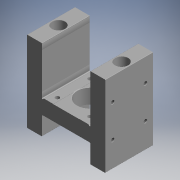
# Autodesk Inventor part: 2608532 EAGF-V2-KF-100---(F)
Saved by Autodesk Inventor 2017.3 (Build 213256000, 256)
## iProperties
Part Number: 2608532 EAGF-V2-KF-100---(F)
Material: Generic
Catalog Web Link: www.cadenas.de
Description: EAGF-(F)-Guide
Vendor: FESTO
Document SubType Name: Modeling
Designer: partserver
Manufacturer: FESTO
Mass: 2427.58 g
Surface Area: 2629 cm^2
Volume: 2427.58 cm^3
Density: 1 g/cm^3
Appearance: PSOLRGB-192-192-192
Category: PARTsolutions
Company: FESTO
Title: 2608532 EAGF-V2-KF-100---(F)
Author: Cadenas PARTsolutions
Comments: Guide
PSOL_IDENT_0: {$CADENAS_DATA\23d-libs\festo\parts\e\eagf\parts\eagf_fuehr.prj},198 {VTYP=3D},{NB=2608532 EAGF-V2-K
PSOL_IDENT_1: F-100---(F)},{LINA=2608532 EAGF-V2-KF-100---(F)},{NN=EAGF-(F)},{DATE=22.07.2021 15:11:35},{GEOMDATE=
PSOL_IDENT_2: 14.04.2021 08:28:38},{VERSION=},{LINEID=30},{WBVAR=},{WBNUMERIC=}  {NB=2608532 EAGF-V2-KF-100---(F)}
PSOL_IDENT_3: ,{LINA=2608532 EAGF-V2-KF-100---(F)},{KT=DUMMY},{TNR=2608532},{TYP=EAGF-V2-KF-100},{KDM=100},{B1=213
PSOL_IDENT_4: .000},{B2=132.000},{B3=70.000},{B4=172.000},{B5=150.000},{D1=35.000},{D2=33.000},{D4=70.000},{D5=18.
PSOL_IDENT_5: 000},{D6=11.000},{D7=10.000},{H1=130.000},{H2=89.000},{H3=65.000},{L1=220.000},{L2=41.000},{L3=128.0
PSOL_IDENT_6: 00},{L4=89.000},{L5=0.000},{L6=24.500},{L7=112.900},{L8=0.000},{T1=0.500},{T2=45.000},{T3=6.000},{T4=
PSOL_IDENT_7: 20.000},{T5=24.000},{F=1.500},{L2J=127.000},{LR1=0.000},{LR2=0.000},{LR3=0.000},{T6=0.000},{LL1=0.00
PSOL_IDENT_8: 0},{LL2=0.000},{LL3=0.000},{LL4=0.000},{LL5=0.000},{TG=89.000}
NB: 2608532 EAGF-V2-KF-100---(F)
NN: EAGF-(F)
NT: Guide
NBSYN: $TNR. $TYP.---(F)
LINA: 2608532 EAGF-V2-KF-100---(F)
CATALOG: Festo
TNR: 2608532
TYP: EAGF-V2-KF-100
KDM: 100
B1: 213
B2: 132
B3: 70
B4: 172
B5: 150
D1: 35
D2: 33
D4: 70
D5: 18
D6: 11
D7: 10
H1: 130
H2: 89
H3: 65
L1: 220
L2: 41
L3: 128
L4: 89
L5: 0
L6: 24.5
L7: 112.9
L8: 0
T1: 0.5
T2: 45
T3: 6
T4: 20
T5: 24
F: 1.5
L2J: 127
LR1: 0
LR2: 0
LR3: 0
T6: 0
LL1: 0
LL2: 0
LL3: 0
LL4: 0
LL5: 0
TG: 89
SUPPLIER: FESTO
ARTICLENO: 2608532 EAGF-V2-KF-100---(F)
BOMINFO: 2608532 EAGF-V2-KF-100---(F)
CREATOR: CADENAS GmbH
Autodesk Inventor part; units mm, degrees
sketch "Sketch_2" plane through (0, 0, 0) normal (0, 1, 0) x (-1, 0, 0)
  arc A0 (106.5, 91) -> (105.5, 92) centre (105.5, 91) ccw
  line L0 (105.5, 92) -> (67, 92)
  arc A1 (67, 92) -> (66, 91) centre (67, 91) ccw
  line L1 (66, 91) -> (66, 43.5)
  arc A2 (63.5, 41) -> (66, 43.5) centre (63.5, 43.5) ccw
  line L2 (63.5, 41) -> (-63.5, 41)
  arc A3 (-66, 43.5) -> (-63.5, 41) centre (-63.5, 43.5) ccw
  line L3 (-66, 43.5) -> (-66, 91)
  arc A4 (-66, 91) -> (-67, 92) centre (-67, 91) ccw
  line L4 (-67, 92) -> (-105.5, 92)
  arc A5 (-105.5, 92) -> (-106.5, 91) centre (-105.5, 91) ccw
  line L5 (-106.5, 91) -> (-106.5, -127)
  arc A6 (-106.5, -127) -> (-105.5, -128) centre (-105.5, -127) ccw
  line L6 (-105.5, -128) -> (-67, -128)
  arc A7 (-67, -128) -> (-66.0931, -126.5786) centre (-67, -127) ccw
  arc A8 (-66.0931, -126.5786) -> (-66, -111.8466) centre (-115.5, -118.9) ccw
  line L7 (-66, -111.8466) -> (-66, -13.0534)
  arc A9 (-66, -13.0534) -> (-65.9994, 1.0491) centre (-115.5, -6) ccw
  arc A10 (-62.0635, 1.5) -> (-65.9994, 1.0491) centre (-64, 1) ccw
  arc A11 (-62.0635, 1.5) -> (-60.127, 0) centre (-60.127, 2) ccw
  line L8 (-60.127, 0) -> (-35, 0)
  line L9 (-35, 0) -> (-35, 0.5)
  line L10 (-35, 0.5) -> (35, 0.5)
  line L11 (35, 0.5) -> (35, 0)
  line L12 (35, 0) -> (60.127, 0)
  arc A12 (60.127, 0) -> (62.0635, 1.5) centre (60.127, 2) ccw
  arc A13 (65.9994, 1.0491) -> (62.0635, 1.5) centre (64, 1) ccw
  arc A14 (65.9994, 1.0491) -> (66, -13.0534) centre (115.5, -6) ccw
  line L13 (66, -13.0534) -> (66, -111.8466)
  arc A15 (66, -111.8466) -> (66.0931, -126.5786) centre (115.5, -118.9) ccw
  arc A16 (66.0931, -126.5786) -> (67, -128) centre (67, -127) ccw
  line L14 (67, -128) -> (105.5, -128)
  arc A17 (105.5, -128) -> (106.5, -127) centre (105.5, -127) ccw
  line L15 (106.5, -127) -> (106.5, 91)
  constraints: 36 point on circle, 32 end point, 18 centre point
extrude "Extrusion1" add sketch "Sketch_2" along normal mid plane 130
sketch "Sketch_3" plane through (0, 0, 0) normal (1, 0, 0) x (0, 1, 0)
  line L0 (0, 0) -> (0, 41)
  line L1 (0, 41) -> (35, 41)
  line L2 (35, 41) -> (35, 1.5)
  line L3 (35, 1.5) -> (36.5, 0)
  line L4 (36.5, 0) -> (0, 0)
  line L5 (0, 0) -> (0, 41)
  constraints: 12 end point
revolve "Revolution1" cut sketch "Sketch_3" angle 360 about axis through (0, 0, 0) along (0, 0, -1)
sketch "Sketch3" plane through (-63.5, 65, 41) normal (0, 0, 1) x (1, 0, 0)
  point P0 (108, -20.5)
hole "Hole1" at (44.5, 44.5, 41) direction (0, 0, -1) diameter 11 depth 41 counterbore diameter 18 counterbore depth 6
pattern_linear "Rectangular Pattern1" count 2 spacing 89 along (-1, 0, 0) count 2 spacing 89 along (0, -1, 0) of "Hole1"
sketch "Sketch_8" plane through (0, 0, 0) normal (0, 1, 0) x (-1, 0, 0)
  line L0 (86, 92) -> (86, -128)
  line L1 (86, -128) -> (68.2321, -128)
  line L2 (68.2321, -128) -> (68.5, -127)
  line L3 (68.5, -127) -> (68.5, -83)
  line L4 (68.5, -83) -> (69.5, -82)
  line L5 (69.5, -82) -> (69.5, 46)
  line L6 (69.5, 46) -> (68.5, 47)
  line L7 (68.5, 47) -> (68.5, 91)
  line L8 (68.5, 91) -> (68.2321, 92)
  line L9 (68.2321, 92) -> (86, 92)
  line L10 (86, 92) -> (86, -128)
  constraints: 22 end point
revolve "Revolution2" cut sketch "Sketch_8" angle 360 about axis through (-86, 0, 92) along (0, 0, 1)
sketch "Sketch_9" plane through (0, 0, 0) normal (0, 1, 0) x (-1, 0, 0)
  line L0 (-86, 92) -> (-86, -128)
  line L1 (-86, -128) -> (-103.7679, -128)
  line L2 (-103.7679, -128) -> (-103.5, -127)
  line L3 (-103.5, -127) -> (-103.5, -83)
  line L4 (-103.5, -83) -> (-102.5, -82)
  line L5 (-102.5, -82) -> (-102.5, 46)
  line L6 (-102.5, 46) -> (-103.5, 47)
  line L7 (-103.5, 47) -> (-103.5, 91)
  line L8 (-103.5, 91) -> (-103.7679, 92)
  line L9 (-103.7679, 92) -> (-86, 92)
  line L10 (-86, 92) -> (-86, -128)
  constraints: 22 end point
revolve "Revolution3" cut sketch "Sketch_9" angle 360 about axis through (86, 0, 92) along (0, 0, 1)
sketch "Sketch6" plane through (0, 65, 0) normal (0, 1, 0) x (1, 0, 0)
  point P0 (75, -24.5)
hole "Hole2" at (75, 65, 24.5) direction (0, -1, 0) diameter 8.376 depth 24 tip angle 120 countersink diameter 10 countersink angle 90 thread size "M10x1.5" class "6H" standard "ISO Metric profile"
pattern_linear "Rectangular Pattern2" count 2 spacing 89 along (0, 0, -1) count 2 spacing 150 along (-1, 0, 0) of "Hole2"
sketch "Sketch7" plane through (-106.5, -65, 91) normal (-1, 0, 0) x (0, 0, 1)
  point P0 (-66.5, 109.5)
hole "Hole3" at (-106.5, 44.5, 24.5) direction (1, 0, 0) diameter 8.376 depth 24 tip angle 120 countersink diameter 10 countersink angle 90 thread size "M10x1.5" class "6H" standard "ISO Metric profile"
pattern_linear "Rectangular Pattern3" count 2 spacing 89 along (0, 0, -1) count 2 spacing 89 along (0, -1, 0) of "Hole3"
sketch "Sketch8" plane through (106.5, -65, -127) normal (1, 0, 0) x (0, 0, -1)
  point P0 (-151.5, 109.5)
hole "Hole4" at (106.5, 44.5, 24.5) direction (-1, 0, 0) diameter 8.376 depth 24 tip angle 120 countersink diameter 10 countersink angle 90 thread size "M10x1.5" class "6H" standard "ISO Metric profile"
pattern_linear "Rectangular Pattern4" count 2 spacing 89 along (0, 0, -1) count 2 spacing 89 along (0, -1, 0) of "Hole4"
ref_plane "ABSTREIF_H_1_XY" through (86, 0, -123.6) normal (0, 0, 1) x (1, 0, 0)
ref_plane "ABSTREIF_H_1_YZ" through (86, 0, -123.6) normal (1, 0, 0) x (0, 1, 0)
ref_plane "ABSTREIF_H_1_ZX" through (86, 0, -123.6) normal (0, 1, 0) x (0, 0, 1)
ref_plane "ABSTREIF_H_2_XY" through (-86, 0, -123.6) normal (0, 0, 1) x (1, 0, 0)
ref_plane "ABSTREIF_H_2_YZ" through (-86, 0, -123.6) normal (1, 0, 0) x (0, 1, 0)
ref_plane "ABSTREIF_H_2_ZX" through (-86, 0, -123.6) normal (0, 1, 0) x (0, 0, 1)
ref_plane "ABSTREIF_V_1_XY" through (86, 0, 87.6) normal (0, 0, -1) x (1, 0, 0)
ref_plane "ABSTREIF_V_1_YZ" through (86, 0, 87.6) normal (1, 0, 0) x (0, -1, 0)
ref_plane "ABSTREIF_V_1_ZX" through (86, 0, 87.6) normal (0, -1, 0) x (0, 0, -1)
ref_plane "ABSTREIF_V_2_XY" through (-86, 0, 87.6) normal (0, 0, -1) x (1, 0, 0)
ref_plane "ABSTREIF_V_2_YZ" through (-86, 0, 87.6) normal (1, 0, 0) x (0, -1, 0)
ref_plane "ABSTREIF_V_2_ZX" through (-86, 0, 87.6) normal (0, -1, 0) x (0, 0, -1)
ref_plane "ANBAU_XY" through (0, 0, 0) normal (0, 0, 1) x (1, 0, 0)
ref_plane "ANBAU_YZ" through (0, 0, 0) normal (1, 0, 0) x (0, 1, 0)
ref_plane "ANBAU_ZX" through (0, 0, 0) normal (0, 1, 0) x (0, 0, 1)
ref_plane "BUSH_H_1_XY" through (86, 0, -123.6) normal (0, 0, -1) x (1, 0, 0)
ref_plane "BUSH_H_1_YZ" through (86, 0, -123.6) normal (1, 0, 0) x (0, -1, 0)
ref_plane "BUSH_H_1_ZX" through (86, 0, -123.6) normal (0, -1, 0) x (0, 0, -1)
ref_plane "BUSH_H_2_XY" through (-86, 0, -123.6) normal (0, 0, -1) x (1, 0, 0)
ref_plane "BUSH_H_2_YZ" through (-86, 0, -123.6) normal (1, 0, 0) x (0, -1, 0)
ref_plane "BUSH_H_2_ZX" through (-86, 0, -123.6) normal (0, -1, 0) x (0, 0, -1)
ref_plane "BUSH_V_1_XY" through (86, 0, 87.6) normal (0, 0, 1) x (1, 0, 0)
ref_plane "BUSH_V_1_YZ" through (86, 0, 87.6) normal (1, 0, 0) x (0, 1, 0)
ref_plane "BUSH_V_1_ZX" through (86, 0, 87.6) normal (0, 1, 0) x (0, 0, 1)
ref_plane "BUSH_V_2_XY" through (-86, 0, 87.6) normal (0, 0, 1) x (1, 0, 0)
ref_plane "BUSH_V_2_YZ" through (-86, 0, 87.6) normal (1, 0, 0) x (0, 1, 0)
ref_plane "BUSH_V_2_ZX" through (-86, 0, 87.6) normal (0, 1, 0) x (0, 0, 1)
ref_plane "DIN912_1_XY" through (44.5, 44.5, 35) normal (0, 0, -1) x (1, 0, 0)
ref_plane "DIN912_1_YZ" through (44.5, 44.5, 35) normal (1, 0, 0) x (0, -1, 0)
ref_plane "DIN912_1_ZX" through (44.5, 44.5, 35) normal (0, -1, 0) x (0, 0, -1)
ref_plane "DIN912_2_XY" through (-44.5, 44.5, 35) normal (0, 0, -1) x (1, 0, 0)
ref_plane "DIN912_2_YZ" through (-44.5, 44.5, 35) normal (1, 0, 0) x (0, -1, 0)
ref_plane "DIN912_2_ZX" through (-44.5, 44.5, 35) normal (0, -1, 0) x (0, 0, -1)
ref_plane "DIN912_3_XY" through (-44.5, -44.5, 35) normal (0, 0, -1) x (1, 0, 0)
ref_plane "DIN912_3_YZ" through (-44.5, -44.5, 35) normal (1, 0, 0) x (0, -1, 0)
ref_plane "DIN912_3_ZX" through (-44.5, -44.5, 35) normal (0, -1, 0) x (0, 0, -1)
ref_plane "DIN912_4_XY" through (44.5, -44.5, 35) normal (0, 0, -1) x (1, 0, 0)
ref_plane "DIN912_4_YZ" through (44.5, -44.5, 35) normal (1, 0, 0) x (0, -1, 0)
ref_plane "DIN912_4_ZX" through (44.5, -44.5, 35) normal (0, -1, 0) x (0, 0, -1)
ref_plane "JOCH_XY" through (0, 0, 127) normal (0, 0, -1) x (1, 0, 0)
ref_plane "JOCH_YZ" through (0, 0, 127) normal (1, 0, 0) x (0, -1, 0)
ref_plane "JOCH_ZX" through (0, 0, 127) normal (0, -1, 0) x (0, 0, -1)
body "Solid1"
